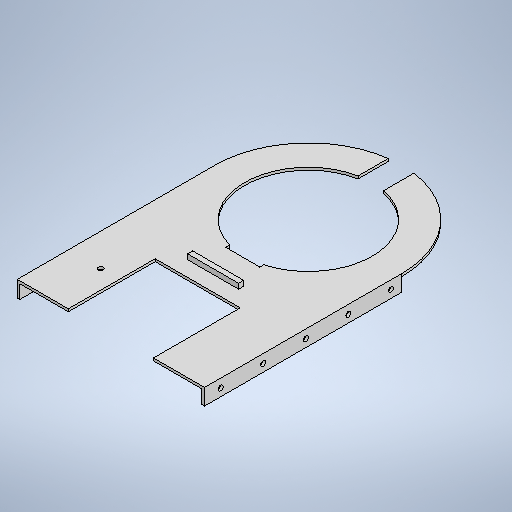
# Autodesk Inventor part: 1 part 06
Saved by Autodesk Inventor 2025 (Build 290162010, 162A)
## iProperties
Created: 2024-07-30
Part Number: 1 part 06
Material: Generisch
Document SubType Name: Modeling
Designer: ffogue
Density: 1 g/cm^3
Appearance: Vorgabe
Author: ffogue
Autodesk Inventor part; units mm, degrees
note: some values were not read from the file. Chosen so that the rebuilt part matches the saved one: direction of "Hole1"; direction of "Hole2".
ref_plane "YZ Plane" through (0, 0, 0) normal (1, 0, 0) x (0, 1, 0)
ref_plane "XZ Plane" through (0, 0, 0) normal (0, 1, 0) x (-1, 0, 0)
ref_plane "XY Plane" through (0, 0, 0) normal (0, 0, 1) x (1, 0, 0)
sketch "Skizze1" plane through (0, 0, 0) normal (0, 0, 1) x (1, 0, 0)
  line L0 (-25, 0) -> (-25, 51)
  line L1 (-25, 51) -> (25, 51)
  line L2 (25, 51) -> (25, 0)
  line L3 (25, 0) -> (55, 0)
  line L4 (55, 0) -> (55, 116)
  arc A0 (55, 116) -> (-55, 116) centre (0, 116) ccw
  line L5 (-55, 116) -> (-55, 0)
  line L6 (-55, 0) -> (-25, 0)
  point P0 (0, 0)
  point P1 (0, 51)
  point P2 (-40, 0)
  dimension "d0" = 25
  dimension "d1" = 51
  dimension "d2" = 116
  dimension "d3" = 55
  constraints: 14 end point, 5 perpendicular, 2 horizontal alignment, 2 midpoint, 2 point on circle, 2 tangent, 2 vertical alignment, 1 centre point, 1 parallel, 1 point on line, 1 vertical
  measures "d0" distance from line of A0.centre L0
  measures "d1" distance between parallel lines of L3 L1
  measures "d2" vertical distance of point (-40, 0) A0.centre
  measures "d3" radius of A0
extrude "Extrusion1" add sketch "Skizze1" along normal mid plane 1.5
sketch "Skizze2" plane through (0, 0, 0.75) normal (0, 0, 1) x (1, 0, 0)
  line L0 (-25, 51) -> (25, 51) projected
  line L1 (25, 51) -> (25, 0) projected
  line L2 (25, 0) -> (55, 0) projected
  line L3 (55, 0) -> (55, 116) projected
  arc A0 (55, 116) -> (-55, 116) centre (0, 116) ccw projected
  line L4 (-55, 116) -> (-55, 0) projected
  line L5 (-55, 0) -> (-25, 0) projected
  line L6 (-25, 0) -> (-25, 51) projected
  circle A1 centre (0, 116) radius 37.5
  point P0 (0, 0)
  dimension "d6" = 75
  constraints: 1 centre point, 1 coincident
  measures "d6" diameter of A1
extrude "Extrusion2" cut sketch "Skizze2" against normal up to surface (1.5 mm away) contours A1
sketch "Skizze3" plane through (0, 0, 0.75) normal (0, 0, 1) x (1, 0, 0)
  arc A0 (55, 116) -> (-55, 116) centre (0, 116) ccw projected
  circle A1 centre (0, 116) radius 37.5 projected
  line L0 (-7.5, 152.7423) -> (-7.5, 170.4862)
  line L1 (7.5, 152.7423) -> (7.5, 170.4862)
  line L2 (0, 116) -> (0, 135.7591) construction
  line L3 (-10, 79.8579) -> (-10, 77.5)
  line L4 (-10, 77.5) -> (10, 77.5)
  line L5 (10, 77.5) -> (10, 79.8579)
  point P0 (0, 0)
  dimension "d9" = 15
  dimension "d12" = 20
  dimension "d13" = 1
  constraints: 12 end point, 6 point on circle, 3 vertical, 2 perpendicular, 1 parallel, 2 other
  measures "d9" distance between parallel lines of L1 L0
  measures "d12" distance between parallel lines of L5 L3
  measures "d13" distance edge to line of A1 L4
extrude "Extrusion3" cut sketch "Skizze3" against normal up to surface (1.5 mm away) contours L1 A1 L0 A0
extrude "Extrusion4" cut sketch "Skizze3" against normal up to surface (1.5 mm away) contours A1 L5 L4 L3
sketch "Skizze5" plane through (0, 0, 0.75) normal (0, 0, 1) x (1, 0, 0)
  line L0 (-15, 63) -> (15, 63)
  line L1 (15, 63) -> (15, 60)
  line L2 (15, 60) -> (-15, 60)
  line L3 (-15, 60) -> (-15, 63)
  point P0 (0, 0)
  point P1 (0, 60)
  dimension "d16" = 3
  dimension "d17" = 30
  dimension "d18" = 60
  constraints: 8 end point, 2 parallel, 1 horizontal, 1 midpoint, 1 perpendicular, 1 vertical alignment
  measures "d16" distance between parallel lines of L2 L0
  measures "d17" distance of L1.end L2.end
  measures "d18" vertical distance of point (0, 0) L1.end
extrude "Extrusion5" add sketch "Skizze5" along normal blind 3
sketch "Sketch9" plane through (55, 0, 0.75) normal (1, 0, 0) x (0, 0, -1)
  line L0 (1.5, 116) -> (1.5, 0) projected
  line L1 (0, 0) -> (0, 116) projected
  line L2 (1.5, 116) -> (0, 116) projected
  line L3 (1.5, 0) -> (0, 0) projected
  line L4 (9.5, 0) -> (9.5, 116)
  line L5 (1.5, 116) -> (1.5, 0)
  line L6 (9.5, 116) -> (0, 116)
  line L7 (0, 0) -> (9.5, 0)
  point P0 (0.75, 0)
  dimension "d39" = 8
  constraints: 8 end point, 2 horizontal, 1 parallel
  measures "d39" distance between parallel lines of L4 L0
extrude "Extrusion7" add sketch "Sketch9" against normal blind 1.5
sketch "Sketch8" plane through (55, 0, 0.75) normal (1, 0, 0) x (0, 0, -1)
  line L0 (0, 0) -> (0, 116) projected
  point P0 (0.75, 0)
  point P1 (5, 109.5)
  point P2 (5, 84.5)
  point P3 (5, 59.5)
  point P4 (5, 34.5)
  point P5 (5, 9.5)
  dimension "d26" = 25
  dimension "d27" = 25
  dimension "d28" = 25
  dimension "d29" = 25
  dimension "d30" = 5
  constraints: 4 vertical alignment
  measures "d26" distance of point (5, 34.5) point (5, 9.5)
  measures "d27" distance of point (5, 59.5) point (5, 34.5)
  measures "d28" distance of point (5, 84.5) point (5, 59.5)
  measures "d29" distance of point (5, 109.5) point (5, 84.5)
  measures "d30" distance from line of L0 point (5, 9.5)
hole "Hole1" at (55, 109.5, -4.25) at (55, 84.5, -4.25) at (55, 59.5, -4.25) at (55, 34.5, -4.25) at (55, 9.5, -4.25) direction (-1, 0, 0) diameter 3 depth 1.5
mirror "Mirror1" about plane through (0, 0, 0) normal (1, 0, 0) of "Hole1", "Extrusion7"
sketch "Sketch10" plane through (0, 0, 0.75) normal (0, 0, 1) x (1, 0, 0)
  line L0 (-55, 0) -> (-25, 0) projected
  line L1 (-55, 116) -> (-55, 0) projected
  point P0 (0, 0)
  point P1 (-36, 30)
  dimension "d42" = 30
  dimension "d43" = 19
  measures "d42" distance from line of L0 point (-36, 30)
  measures "d43" distance from line of point (-36, 30) L1
hole "Hole2" at (-36, 30, 0.75) direction (0, 0, -1) diameter 3 depth 1.5
equation "\"d27\" = d26"
equation "\"d28\" = d26"
equation "\"d29\" = d26"
